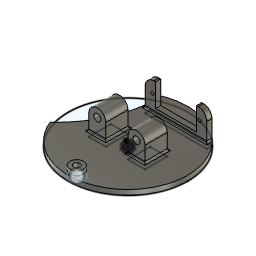
ctr fusion 3d model (Autodesk Fusion 360 archive; units mm, degrees)
design "disk"
Autodesk Fusion 360 part; units mm, degrees
sketch "Sketch1" plane through (0, 0, 0) normal (0, 0, 1) x (1, 0, 0)
  circle A0 centre (0, 0) radius 35
  circle A1 centre (0, 0) radius 1.85
  line L0 (-11.9, 25) -> (24.25, 25)
  line L1 (24.25, 25) -> (24.25, 22)
  line L2 (24.25, 22) -> (-11.9, 22)
  line L3 (-11.9, 22) -> (-11.9, 25)
  circle A2 centre (0, -30) radius 1.85
  circle A3 centre (0, -30) radius 4
  line L4 (-16.5, 6.49) -> (-6.5, 6.49)
  line L5 (-6.5, 6.49) -> (-6.5, -6.49)
  line L6 (-6.5, -6.49) -> (-16.5, -6.49)
  line L7 (-16.5, -6.49) -> (-16.5, 6.49)
  line L8 (6.5, 6.49) -> (16.5, 6.49)
  line L9 (16.5, 6.49) -> (16.5, -6.49)
  line L10 (16.5, -6.49) -> (6.5, -6.49)
  line L11 (6.5, -6.49) -> (6.5, 6.49)
  dimension "d1" = 70
  dimension "d2" = 3.7
  dimension "d3" = 25
  dimension "d4" = 3
  dimension "d5" = 36.15
  dimension "d6" = 11.9
  dimension "d7" = 30
  dimension "d8" = 8
  dimension "d9" = 3.7
  dimension "d10" = 6.5
  dimension "d11" = 6.5
  dimension "d12" = 10
  dimension "d13" = 10
  dimension "d14" = 12.98
  dimension "d15" = 12.98
  dimension "d16" = 6.49
  dimension "d17" = 6.49
  constraint coincident A0.centre A1.centre
  constraint horizontal L0
  constraint vertical L1
  constraint horizontal L2
  constraint vertical L3
  constraint concentric A2 A3
  constraint horizontal L4
  constraint vertical L5
  constraint horizontal L6
  constraint vertical L7
  constraint horizontal L8
  constraint vertical L9
  constraint horizontal L10
  constraint vertical L11
  measures "d1" diameter of A0
  measures "d2" diameter of A1
  measures "d3" distance of A0.centre L0
  measures "d4" distance of L0.start L2.end
  measures "d5" distance of L1.end L2.end
  measures "d6" distance of A0.centre L3
  measures "d7" distance of A0.centre A2.centre
  measures "d8" diameter of A3
  measures "d9" diameter of A2
  measures "d10" distance of A0.centre L5
  measures "d11" distance of A0.centre L11
  measures "d12" distance of L9.end L10.end
  measures "d13" distance of L5.end L6.end
  measures "d14" distance of L4.start L6.end
  measures "d15" distance of L8.end L9.end
  measures "d16" distance of A0.centre L8
  measures "d17" distance of A0.centre L4
extrude "Extrude1" add sketch "Sketch1" along normal blind 3 contours A0
extrude "Extrude2" add sketch "Sketch1" along normal blind 5.6 contours A3
extrude "Extrude3" add sketch "Sketch1" along normal blind 17.25 contours L4 L5 L6 L7 | L8 L9 L10 L11
extrude "Extrude4" add sketch "Sketch1" along normal blind 19 contours L0 L1 L2 L3
sketch "Sketch2" plane through (0, 25, 0) normal (0, 1, 0) x (-1, 0, 0)
  line L0 (-24.25, 3) -> (11.9, 3)
  line L1 (11.9, 3) -> (11.9, 19)
  line L2 (11.9, 19) -> (-24.25, 19)
  line L3 (-24.25, 19) -> (-24.25, 3)
  line L4 (-18.175, 19) -> (5.825, 19)
  line L5 (5.825, 19) -> (5.825, 5.5)
  line L6 (5.825, 5.5) -> (-18.175, 5.5)
  line L7 (-18.175, 5.5) -> (-18.175, 19)
  circle A0 centre (7.675, 12.25) radius 0.9
  circle A1 centre (-20.025, 12.25) radius 0.9
  dimension "d26" = 24
  dimension "d27" = 13.5
  dimension "d28" = 1.8
  dimension "d29" = 1.8
  dimension "d30" = 6.75
  dimension "d31" = 6.75
  dimension "d32" = 6.075
  dimension "d33" = 6.075
  dimension "d35" = 1.85
  dimension "d37" = 1.85
  constraint horizontal L4
  constraint vertical L5
  constraint horizontal L6
  constraint vertical L7
  constraint coincident L2 L4.start
  measures "d26" distance of L5.end L6.end
  measures "d27" distance of L4.end L5.end
  measures "d28" diameter of A1
  measures "d29" diameter of A0
  measures "d30" distance of L2 A0.centre
  measures "d31" distance of L4 A1.centre
  measures "d32" distance of L1 L5
  measures "d33" distance of L3 L7
  measures "d35" distance of L5 A0.centre
  measures "d37" distance of L7 A1.centre
sketch "Sketch4" plane through (0, -6.49, 0) normal (0, -1, 0) x (1, 0, 0)
  line L0 (6.5, 3) -> (16.5, 3)
  line L1 (16.5, 3) -> (16.5, 17.25)
  line L2 (16.5, 17.25) -> (6.5, 17.25)
  line L3 (6.5, 17.25) -> (6.5, 3)
  circle A0 centre (11.5, 12.25) radius 2.1
  circle A1 centre (-11.5, 12.25) radius 2.1
  line L4 (-6.5, 3) -> (-6.5, 17.25)
  line L5 (-16.5, 17.25) -> (-6.5, 17.25)
  dimension "d38" = 4.2
  dimension "d39" = 4.2
  dimension "d40" = 5
  dimension "d41" = 5
  dimension "d42" = 5
  dimension "d43" = 5
  measures "d38" diameter of A0
  measures "d39" diameter of A1
  measures "d40" distance of A1.centre L4
  measures "d41" distance of L3 A0.centre
  measures "d42" distance of L2 A0.centre
  measures "d43" distance of A1.centre L5
extrude "Extrude5" cut sketch "Sketch4" along normal blind 0 and the other way blind 13 contours A0 | A1
extrude "Extrude6" cut sketch "Sketch2" along normal blind 0 and the other way blind 3 contours L2 L4 L5 L6 L7 | A0 | A1
fillet "Fillet1" radius 5 6 edges at (-16.5, 0, 17.25) (-6.5, 0, 17.25) (6.5, 0, 17.25) (16.5, 0, 17.25) (-11.9, 23.5, 19) (24.25, 23.5, 19)
sketch "Sketch5" plane through (0, 0, 3) normal (0, 0, 1) x (-1, 0, 0)
  circle A0 centre (0, 30) radius 4
  circle A1 centre (0, 0) radius 1.85
  circle A2 centre (72.6886, -31.0318) radius 60
  circle A3 centre (0, 0) radius 35
  line L0 (-24.25, -22) -> (11.9, -22)
  line L1 (11.9, -22) -> (11.9, -25)
  line L2 (11.9, -25) -> (-24.25, -25)
  line L3 (-24.25, -25) -> (-24.25, -22)
  line L4 (6.5, 6.49) -> (16.5, 6.49)
  line L5 (16.5, 6.49) -> (16.5, -6.49)
  line L6 (16.5, -6.49) -> (6.5, -6.49)
  line L7 (6.5, -6.49) -> (6.5, 6.49)
  line L8 (-16.5, 6.49) -> (-6.5, 6.49)
  line L9 (-6.5, 6.49) -> (-6.5, -6.49)
  line L10 (-6.5, -6.49) -> (-16.5, -6.49)
  line L11 (-16.5, -6.49) -> (-16.5, 6.49)
  circle A4 centre (0, 0) radius 35
  dimension "d60" = 120
  measures "d60" diameter of A2
extrude "Extrude7" cut sketch "Sketch5" along normal blind 0 and the other way blind 3 contours A2 A3 A4 picked at (24.1272, -5.8822)
fillet "Fillet3" radius 1 12 edges at (-6.5, 0, 3) (-11.5, -6.49, 3) (11.5, -6.49, 3) (16.5, 0, 3) (6.175, 22, 3) (6.5, 0, 3) (11.5, 6.49, 3) (-11.5, 6.49, 3) (-16.5, 0, 3) (6.175, 25, 3) (-11.9, 23.5, 3) (24.25, 23.5, 3)

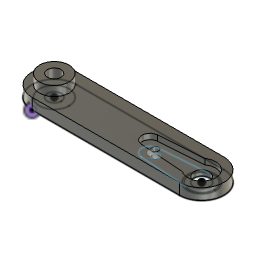
design "servo arm base"
Autodesk Fusion 360 part; units mm, degrees
sketch "Sketch1" plane through (0, 0, 0) normal (0, 0, 1) x (1, 0, 0)
  line L0 (0, 0) -> (40, 0)
  line L1 (40, 12) -> (0, 12)
  arc A0 (0, 12) -> (0, 0) centre (0, 6) ccw
  arc A1 (40, 0) -> (40, 12) centre (40, 6) ccw
  circle A2 centre (40, 6) radius 3.78
  circle A3 centre (40, 6) radius 2.1
  circle A4 centre (0, 6) radius 4
  circle A5 centre (0, 6) radius 1.85
  circle A6 centre (27.4, 6) radius 0.9
  circle A7 centre (40, 6) radius 3.38
  line L2 (38.7491, 2.86) -> (25.8392, 3.8059)
  line L3 (38.7491, 9.14) -> (25.8392, 8.1941)
  arc A8 (25.8392, 8.1941) -> (25.8392, 3.8059) centre (26, 6) ccw
  dimension "d1" = 40
  dimension "d2" = 12
  dimension "d3" = 7.56
  dimension "d4" = 4.2
  dimension "d5" = 8
  dimension "d6" = 3.7
  dimension "d7" = 12.6
  dimension "d9" = 14
  dimension "d10" = 1.8
  dimension "d11" = 6
  dimension "d12" = 6.76
  dimension "d13" = 2.86
  dimension "d14" = 2.86
  dimension "d15" = 6.28
  dimension "d22" = 1.4
  dimension "d23" = 2.2
  constraint horizontal L0
  constraint horizontal L1
  constraint coincident L0.start A0.end
  constraint coincident L0.start A0
  constraint coincident L0 A0.end
  constraint concentric A1 A2
  constraint concentric A1 A3
  constraint concentric A0 A4
  constraint concentric A0 A5
  constraint concentric A1 A7
  constraint coincident A7 L2.start
  constraint coincident A7 L3.start
  measures "d1" distance of L1.start L1.end
  measures "d2" distance of L0.start L1.end
  measures "d3" diameter of A2
  measures "d4" diameter of A3
  measures "d5" diameter of A4
  measures "d6" diameter of A5
  measures "d7" distance of A1.centre A6.centre
  measures "d9" distance of A1.centre A8.centre
  measures "d10" diameter of A6
  measures "d11" distance of L1.start A1.centre
  measures "d12" diameter of A7
  measures "d13" distance of L1 L3.start
  measures "d14" distance of L0 L2.start
  measures "d15" distance of L2.start L3.start
  measures "d22" distance of A6.centre A8.centre
  measures "d23" radius of A8
extrude "Extrude1" add sketch "Sketch1" along normal blind 3 contours L0 L1 A0 A1
extrude "Extrude2" add sketch "Sketch1" along normal blind 5.6 contours A4
extrude "Extrude3" add sketch "Sketch1" along normal blind 1.5 contours A2 A7 L2 L3 | A2 A7 L2 L3 | A2 L2 L3 A8 | A7

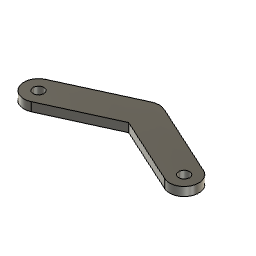
design "base arm"
Autodesk Fusion 360 part; units mm, degrees
sketch "Sketch1" plane through (0, 0, 0) normal (0, 0, 1) x (1, 0, 0)
  circle A0 centre (0, 5) radius 1.85
  circle A1 centre (50, 5) radius 1.85
  line L0 (49.986, 5.0064) -> (50, 5)
  line L1 (27.083, 21.0019) -> (52.083, 9.5455)
  line L2 (22.917, 21.0019) -> (-2.083, 9.5455)
  line L3 (25, 10.9564) -> (2.083, 0.4545)
  line L4 (25, 10.9564) -> (47.8891, 0.4674)
  arc A2 (27.083, 21.0019) -> (22.917, 21.0019) centre (25, 16.4564) ccw
  arc A3 (-2.083, 9.5455) -> (2.083, 0.4545) centre (0, 5) ccw
  arc A4 (47.8891, 0.4674) -> (52.083, 9.5455) centre (50, 5) ccw
  dimension "d3" = 3.7
  dimension "d4" = 3.7
  dimension "d9" = 50
  dimension "d10" = 27.5
  dimension "d11" = 27.5
  dimension "d14" = 25
  dimension "d17" = 5
  dimension "d18" = 5
  dimension "d21" = 130.76
  constraint concentric A0 A3
  constraint coincident origin A3
  constraint coincident A1.centre L0.end
  measures "d3" diameter of A0
  measures "d4" diameter of A1
  measures "d9" distance of A0.centre A1.centre
  measures "d10" distance of A0.centre A2.centre
  measures "d11" distance of A1.centre A2.centre
  measures "d14" horizontal distance of A0.centre A2.centre
  measures "d17" distance of L2.start A2.centre
  measures "d18" distance of L1.start A2.centre
  measures "d21" angle of L3 L4
extrude "Extrude2" add sketch "Sketch1" along normal blind 3

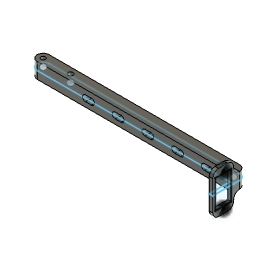
design "rod arm"
Autodesk Fusion 360 part; units mm, degrees
sketch "Sketch1" plane through (0, 0, 0) normal (0, 0, 1) x (1, 0, 0)
  line L0 (5, 0) -> (170, 0)
  line L1 (170, 0) -> (170, 5)
  line L2 (165, 10) -> (5, 10)
  circle A0 centre (5, 5) radius 1.85
  circle A1 centre (28, 5) radius 2.1
  line L3 (170, 0) -> (167, 0)
  line L4 (167, 0) -> (167, -17.5)
  line L5 (167, -17.5) -> (170, -17.5)
  line L6 (170, -17.5) -> (170, 0)
  arc A2 (5, 10) -> (5, 0) centre (5, 5) ccw
  arc A3 (170, 5) -> (165, 10) centre (165, 5) ccw
  dimension "d3" = 10
  dimension "d4" = 10
  dimension "d5" = 5
  dimension "d7" = 5
  dimension "d8" = 5
  dimension "d9" = 4.2
  dimension "d10" = 3.7
  dimension "d11" = 5
  dimension "d12" = 23
  dimension "d13" = 3
  dimension "d14" = 17.5
  dimension "d15" = 160
  dimension "d16" = 10
  constraint horizontal L0
  constraint vertical L1
  constraint horizontal L2
  constraint concentric A0 A2
  constraint horizontal L3
  constraint vertical L4
  constraint horizontal L5
  constraint vertical L6
  measures "d3" diameter of A2
  measures "d4" diameter of A3
  measures "d5" distance of L0 A0.centre
  measures "d7" distance of L1 A3.centre
  measures "d8" distance of L0 A3.centre
  measures "d9" diameter of A1
  measures "d10" diameter of A0
  measures "d11" distance of L2 A1.centre
  measures "d12" distance of A0.centre A1.centre
  measures "d13" distance of L4 L6
  measures "d14" distance of L0.end L5.end
  measures "d15" distance of L2.end L2.start
  measures "d16" distance of L0 L2
extrude "Extrude1" add sketch "Sketch1" along normal mid plane 12.98 contours L0 L1 L2 L3 A2 A3
extrude "Extrude2" add sketch "Sketch1" along normal mid plane 35 contours L0 L3 L4 L5 L6
sketch "Sketch2" plane through (170, 0, 0) normal (1, 0, 0) x (0, 1, 0)
  line L0 (5, -6.49) -> (5, 6.49)
  line L1 (5, 6.49) -> (0, 6.49)
  line L2 (0, 6.49) -> (0, 17.5)
  line L3 (0, 17.5) -> (-17.5, 17.5)
  line L4 (-17.5, 17.5) -> (-17.5, -17.5)
  line L5 (-17.5, -17.5) -> (0, -17.5)
  line L6 (0, -17.5) -> (0, -6.49)
  line L7 (0, -6.49) -> (5, -6.49)
  line L8 (-2, 12) -> (-15.5, 12)
  line L9 (-15.5, 12) -> (-15.5, -12)
  line L10 (-15.5, -12) -> (-2, -12)
  line L11 (-2, -12) -> (-2, 12)
  circle A0 centre (-8.75, 13.85) radius 0.85
  circle A1 centre (-8.75, -13.85) radius 0.85
  dimension "d21" = 24
  dimension "d22" = 13.5
  dimension "d23" = 2
  dimension "d24" = 5.5
  dimension "d25" = 2
  dimension "d26" = 5.5
  dimension "d27" = 1.7
  dimension "d28" = 1.7
  dimension "d29" = 8.75
  dimension "d30" = 8.75
  dimension "d31" = 1.85
  dimension "d32" = 1.85
  constraint horizontal L8
  constraint vertical L9
  constraint horizontal L10
  constraint vertical L11
  measures "d21" distance of L8.end L9.end
  measures "d22" distance of L9 L11
  measures "d23" distance of L4 L9
  measures "d24" distance of L3 L8
  measures "d25" distance of L6 L11
  measures "d26" distance of L5 L10
  measures "d27" diameter of A1
  measures "d28" diameter of A0
  measures "d29" distance of L2 A0.centre
  measures "d30" distance of L6 A1.centre
  measures "d31" distance of L10 A1.centre
  measures "d32" distance of L8 A0.centre
extrude "Extrude3" cut sketch "Sketch2" against normal blind 3 contours L8 L9 L10 L11 | A0 | A1
fillet "Fillet1" radius 5 2 edges at (168.5, 0, 6.49) (168.5, 0, -6.49)
fillet "Fillet2" radius 5 4 edges at (168.5, 0, -17.5) (168.5, 0, 17.5) (168.5, -17.5, 17.5) (168.5, -17.5, -17.5)
fillet "Fillet3" radius 2.5 2 edges at (167, 2.5, 6.49) (167, 2.5, -6.49)
fillet "Fillet4" radius 1 1 edges at (167, 0, 0)
sketch "Sketch3" plane through (0, 0, 0) normal (0, -1, 0) x (1, 0, 0)
  line L0 (166, -6.99) -> (166, 6.99)
  arc A0 (164.5, 6.49) -> (166, 6.99) centre (164.5, 8.99) ccw
  line L1 (164.5, 6.49) -> (5, 6.49)
  line L2 (5, 6.49) -> (5, -6.49)
  line L3 (5, -6.49) -> (164.5, -6.49)
  arc A1 (166, -6.99) -> (164.5, -6.49) centre (164.5, -8.99) ccw
  line L4 (45.5, 2.5) -> (50.5, 2.5)
  line L5 (50.5, -2.5) -> (45.5, -2.5)
  line L6 (70.5, 2.5) -> (75.5, 2.5)
  line L7 (75.5, -2.5) -> (70.5, -2.5)
  line L8 (95.5, 2.5) -> (100.5, 2.5)
  line L9 (100.5, -2.5) -> (95.5, -2.5)
  line L10 (120.5, 2.5) -> (125.5, 2.5)
  line L11 (125.5, -2.5) -> (120.5, -2.5)
  line L12 (145.5, 2.5) -> (150.5, 2.5)
  line L13 (150.5, -2.5) -> (145.5, -2.5)
  arc A2 (45.5, 2.5) -> (43, 0) centre (45.5, 0) ccw
  arc A3 (43, 0) -> (45.5, -2.5) centre (45.5, 0) ccw
  arc A4 (53, 0) -> (50.5, 2.5) centre (50.5, 0) ccw
  arc A5 (50.5, -2.5) -> (53, 0) centre (50.5, 0) ccw
  arc A6 (70.5, 2.5) -> (68, 0) centre (70.5, 0) ccw
  arc A7 (78, 0) -> (75.5, 2.5) centre (75.5, 0) ccw
  arc A8 (75.5, -2.5) -> (78, 0) centre (75.5, 0) ccw
  arc A9 (68, 0) -> (70.5, -2.5) centre (70.5, 0) ccw
  arc A10 (95.5, 2.5) -> (93, 0) centre (95.5, 0) ccw
  arc A11 (93, 0) -> (95.5, -2.5) centre (95.5, 0) ccw
  arc A12 (103, 0) -> (100.5, 2.5) centre (100.5, 0) ccw
  arc A13 (100.5, -2.5) -> (103, 0) centre (100.5, 0) ccw
  arc A14 (120.5, 2.5) -> (118, 0) centre (120.5, 0) ccw
  arc A15 (118, 0) -> (120.5, -2.5) centre (120.5, 0) ccw
  arc A16 (128, 0) -> (125.5, 2.5) centre (125.5, 0) ccw
  arc A17 (125.5, -2.5) -> (128, 0) centre (125.5, 0) ccw
  arc A18 (145.5, 2.5) -> (143, 0) centre (145.5, 0) ccw
  arc A19 (143, 0) -> (145.5, -2.5) centre (145.5, 0) ccw
  arc A20 (150.5, -2.5) -> (153, 0) centre (150.5, 0) ccw
  arc A21 (153, 0) -> (150.5, 2.5) centre (150.5, 0) ccw
  point P0 (43, 2.5)
  point P1 (53, 2.5)
  point P2 (53, -2.5)
  point P3 (28, 0)
  dimension "d43" = 10
  dimension "d44" = 5
  dimension "d45" = 3.99
  dimension "d51" = 2.5
  dimension "d52" = 2.5
  dimension "d53" = 2.5
  constraint horizontal L4
  constraint horizontal L5
  constraint coincident P0 L4
  constraint tangent L4 A2
  constraint tangent L5 A3
  constraint equal A2 A3
  constraint coincident A2.end A3.start
  constraint coincident P1 L4
  constraint tangent L4 A4
  constraint equal A2 A4
  constraint coincident P2 L5
  constraint tangent L5 A5
  constraint equal A2 A5
  constraint coincident A4.start A5.end
  constraint tangent L6 A6
  constraint tangent L6 A7
  constraint tangent L7 A8
  constraint equal A7 A8
  constraint coincident A7.start A8.end
  constraint tangent L7 A9
  constraint equal A7 A9
  constraint coincident A6.end A9.start
  constraint tangent L8 A10
  constraint equal A7 A10
  constraint tangent L9 A11
  constraint equal A7 A11
  constraint coincident A10.end A11.start
  constraint tangent L8 A12
  constraint equal A7 A12
  constraint tangent L9 A13
  constraint equal A7 A13
  constraint coincident A12.start A13.end
  constraint tangent L10 A14
  constraint equal A7 A14
  constraint tangent L11 A15
  constraint equal A7 A15
  constraint coincident A14.end A15.start
  constraint tangent L10 A16
  constraint equal A7 A16
  constraint tangent L11 A17
  constraint equal A7 A17
  constraint coincident A16.start A17.end
  constraint tangent L12 A18
  constraint equal A7 A18
  constraint tangent L13 A19
  constraint equal A7 A19
  constraint coincident A18.end A19.start
  constraint tangent L13 A20
  constraint equal A7 A20
  constraint tangent L12 A21
  constraint equal A7 A21
  constraint coincident A20.end A21.start
  measures "d43" distance of P0 P1
  measures "d44" distance of P1 P2
  measures "d45" distance of L1 L4
  measures "d51" radius of A2
  measures "d52" radius of A6
  measures "d53" radius of A7
extrude "Extrude4" cut sketch "Sketch3" against normal blind 10 contours L4 L5 A2 A3 A4 A5 | L6 L7 A6 A7 A8 A9 | L8 L9 A10 A11 A12 A13 | L10 L11 A14 A15 A16 A17 | L12 L13 A18 A19 A20 A21

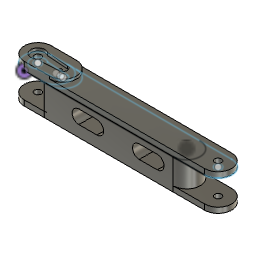
design "servo arm"
Autodesk Fusion 360 part; units mm, degrees
sketch "Sketch1" plane through (0, 0, 0) normal (0, 0, 1) x (1, 0, 0)
  line L0 (0, 0) -> (100, 0)
  line L1 (100, 15) -> (0, 15)
  arc A0 (0, 15) -> (0, 0) centre (0, 7.5) ccw
  arc A1 (100, 0) -> (100, 15) centre (100, 7.5) ccw
  circle A2 centre (0, 7.5) radius 1.85
  arc A3 (14, 0) -> (14, 15) centre (14, 7.5) ccw
  arc A4 (9, 0) -> (9, 15) centre (10, 7.5) ccw
  circle A5 centre (12.6, 7.5) radius 0.8
  line L2 (2.2313, 10.6742) -> (14.1692, 9.7938)
  line L3 (2.2313, 4.3258) -> (14.1692, 5.2062)
  arc A6 (2.2313, 10.6742) -> (2.2313, 4.3258) centre (0, 7.5) ccw
  arc A7 (14.1692, 5.2062) -> (14.1692, 9.7938) centre (14, 7.5) ccw
  arc A8 (82.5, 0) -> (82.5, 15) centre (82.5, 7.5) ccw
  circle A9 centre (100, 7.5) radius 1.85
  dimension "d3" = 100
  dimension "d4" = 15
  dimension "d5" = 3.7
  dimension "d6" = 7.5
  dimension "d7" = 15
  dimension "d8" = 14
  dimension "d9" = 7.76
  dimension "d12" = 4.6
  dimension "d14" = 1.4
  dimension "d16" = 1.6
  dimension "d17" = 4.3258
  dimension "d18" = 4.3258
  dimension "d19" = 6.3484
  dimension "d20" = 10
  dimension "d22" = 17.5
  dimension "d23" = 7.5
  dimension "d24" = 3.7
  dimension "d74" = 3.88
  constraint horizontal L0
  constraint horizontal L1
  constraint coincident L0.start A0.end
  constraint coincident L0.start A0
  constraint coincident L0 A0.end
  constraint concentric A0 A2
  constraint concentric A0 A6
  constraint tangent L0 A3
  constraint coincident L1 A3.end
  constraint coincident L0 A3.start
  constraint concentric A3 A7
  constraint coincident L1 A4.end
  constraint coincident L0 A4.start
  constraint tangent L2 A7
  constraint tangent L3 A7
  constraint tangent L0 A8
  constraint coincident L1 A8.end
  constraint coincident L0 A8.start
  constraint concentric A1 A9
  measures "d3" distance of L1.start L1.end
  measures "d4" distance of L0.start L1.end
  measures "d5" diameter of A2
  measures "d6" radius of A0
  measures "d7" diameter of A3
  measures "d8" distance of A0.centre A3.centre
  measures "d9" diameter of A6
  measures "d12" diameter of A7
  measures "d14" distance of A3.centre A5.centre
  measures "d16" diameter of A5
  measures "d17" distance of L1 L2.start
  measures "d18" distance of L0 L3.start
  measures "d19" distance of L2.start L3.start
  measures "d20" distance of A0.centre A4.centre
  measures "d22" distance of A1.centre A8.centre
  measures "d23" radius of A8
  measures "d24" diameter of A9
  measures "d74" radius of A6
extrude "Extrude1" add sketch "Sketch1" along normal blind 4.5 contours L0 L1 A0 A4 | L0 L1 A3 A4 makes body 1
extrude "Extrude2" add sketch "Sketch1" along normal blind 3 contours L0 L1 A3 A8 | L0 L1 A1 A8 | L2 L3 A6 A7 bodies 1
extrude "Extrude3" add sketch "Sketch1" along normal blind 0 and the other way blind 17 contours L0 L1 A3 A4 | L0 L1 A3 A8 bodies 1
extrude "Extrude4" add sketch "Sketch1" against normal blind 3 from surface at -14 separate body contours L0 L1 A0 A4 | L0 L1 A1 A8 | A5 | L2 L3 A6 A7 makes body 2 at (96.0418, 11.3328, -14) makes body 3 at (7.95, 7.5, -14)
sketch "Sketch4" plane through (0, 15, 0) normal (0, 1, 0) x (-1, 0, 0)
  line L0 (-100, 0) -> (-82.5, 0)
  line L1 (-82.5, 0) -> (-82.5, -17)
  line L2 (-82.5, -17) -> (-11, -17)
  line L3 (-11, -17) -> (-11, 0)
  line L4 (-11, 0) -> (0, 0)
  line L5 (0, 0) -> (0, 4.5)
  line L6 (0, 4.5) -> (-14, 4.5)
  line L7 (-14, 4.5) -> (-14, 3)
  line L8 (-14, 3) -> (-100, 3)
  line L9 (-100, 3) -> (-100, 0)
  line L10 (-30.25, -10.75) -> (-40.25, -10.75)
  line L11 (-40.25, -3.25) -> (-30.25, -3.25)
  line L12 (-63.75, -10.75) -> (-73.75, -10.75)
  line L13 (-73.75, -3.25) -> (-63.75, -3.25)
  arc A0 (-30.25, -10.75) -> (-26.5, -7) centre (-30.25, -7) ccw
  arc A1 (-26.5, -7) -> (-30.25, -3.25) centre (-30.25, -7) ccw
  arc A2 (-40.25, -3.25) -> (-44, -7) centre (-40.25, -7) ccw
  arc A3 (-44, -7) -> (-40.25, -10.75) centre (-40.25, -7) ccw
  arc A4 (-63.75, -10.75) -> (-60, -7) centre (-63.75, -7) ccw
  arc A5 (-60, -7) -> (-63.75, -3.25) centre (-63.75, -7) ccw
  arc A6 (-73.75, -3.25) -> (-77.5, -7) centre (-73.75, -7) ccw
  arc A7 (-77.5, -7) -> (-73.75, -10.75) centre (-73.75, -7) ccw
  point P0 (-26.5, -10.75)
  point P1 (-44, -10.75)
  point P2 (-44, -3.25)
  point P3 (-60, -10.75)
  point P4 (-77.5, -10.75)
  point P5 (-60, -3.25)
  dimension "d60" = 7.5
  dimension "d61" = 17.5
  dimension "d62" = 6.25
  dimension "d63" = 6.25
  dimension "d65" = 7.5
  dimension "d66" = 17.5
  dimension "d67" = 6.25
  dimension "d68" = 6.25
  dimension "d71" = 3.75
  constraint horizontal L10
  constraint horizontal L11
  constraint horizontal L12
  constraint horizontal L13
  constraint coincident P0 L10
  constraint tangent L10 A0
  constraint tangent L11 A1
  constraint equal A0 A1
  constraint coincident A0.end A1.start
  constraint coincident P2 L11
  constraint tangent L11 A2
  constraint equal A0 A2
  constraint coincident P1 L10
  constraint tangent L10 A3
  constraint equal A0 A3
  constraint coincident A2.end A3.start
  constraint coincident P3 L12
  constraint tangent L12 A4
  constraint equal A0 A4
  constraint coincident P5 L13
  constraint tangent L13 A5
  constraint equal A0 A5
  constraint coincident A4.end A5.start
  constraint tangent L13 A6
  constraint equal A0 A6
  constraint coincident P4 L12
  constraint tangent L12 A7
  constraint equal A0 A7
  constraint coincident A6.end A7.start
  measures "d60" distance of P1 P2
  measures "d61" distance of P0 P1
  measures "d62" distance of L2 L10
  measures "d63" distance of L8 L11
  measures "d65" distance of P3 P5
  measures "d66" distance of P3 P4
  measures "d67" distance of L2 L12
  measures "d68" distance of L8 L13
  measures "d71" radius of A0
extrude "Extrude6" cut sketch "Sketch4" against normal blind 15 contours L10 L11 A0 A1 A2 A3 | L12 L13 A4 A5 A6 A7 bodies 1
